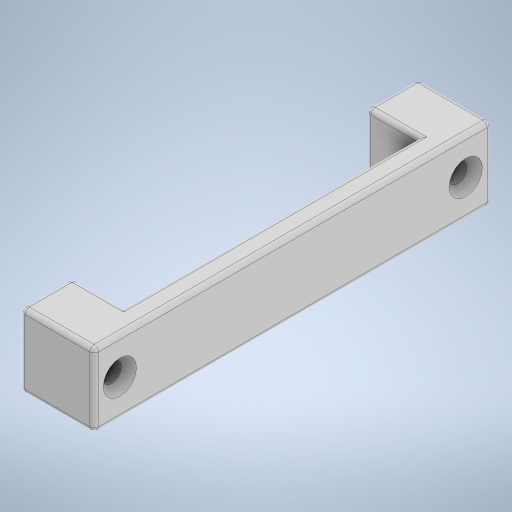
# Autodesk Inventor part: PMSretainer
Saved by Autodesk Inventor 2024 (Build 280153000, 153)
## iProperties
Created: 2023-11-03
Part Number: PMSretainer
Material: Generic
Document SubType Name: Modeling
Designer: njspada
Density: 1 g/cm^3
Appearance: Default
Author: njspada
Autodesk Inventor part; units mm, degrees
ref_plane "YZ Plane" through (0, 0, 0) normal (1, 0, 0) x (0, 1, 0)
ref_plane "XZ Plane" through (0, 0, 0) normal (0, 1, 0) x (-1, 0, 0)
ref_plane "XY Plane" through (0, 0, 0) normal (0, 0, 1) x (1, 0, 0)
sketch "Sketch1" plane through (0, 0, 0) normal (0, 1, 0) x (-1, 0, 0)
  line L0 (0, 0) -> (3.81, 0)
  line L1 (3.81, 0) -> (3.81, -50.8)
  line L2 (3.81, -50.8) -> (0, -50.8)
  line L3 (0, -50.8) -> (0, 0)
  line L4 (0, 0) -> (12.7, 0)
  line L5 (12.7, 0) -> (12.7, 8.89)
  line L6 (12.7, 8.89) -> (0, 8.89)
  line L7 (0, 8.89) -> (0, 0)
  line L8 (0, -50.8) -> (12.7, -50.8)
  line L9 (12.7, -50.8) -> (12.7, -59.69)
  line L10 (12.7, -59.69) -> (0, -59.69)
  line L11 (0, -59.69) -> (0, -50.8)
  dimension "d0" = 3.81
  dimension "d1" = 50.8
  dimension "d2" = 12.7
  dimension "d3" = 8.89
  dimension "d4" = 12.7
  dimension "d5" = 8.89
  constraints: 24 end point, 6 parallel, 3 horizontal, 3 perpendicular
  measures "d0" distance of L1.end L2.end
  measures "d1" distance of L0.end L1.end
  measures "d2" distance of L6.end L5.end
  measures "d3" distance of L5.end L4.end
  measures "d4" distance of L9.end L10.end
  measures "d5" distance of L8.end L9.end
extrude "Extrusion1" add sketch "Sketch1" along normal blind 12.7
sketch "Sketch2" plane through (0, 0, 8.89) normal (1, 0, 0) x (0, 0, -1)
  line L0 (0, 12.7) -> (68.58, 12.7) construction
  line L1 (8.89, 0) -> (0, 0) construction
  line L2 (0, 0) -> (0, 12.7) construction
  line L3 (0, 12.7) -> (8.89, 12.7) construction
  line L4 (8.89, 12.7) -> (8.89, 0) construction
  line L5 (34.29, 12.7) -> (34.29, 0) construction
  line L6 (59.69, 0) -> (8.89, 0) construction
  point P0 (4.445, 6.35)
  point P1 (64.135, 6.35)
  constraints: 10 end point, 2 midpoint, 2 parallel, 1 horizontal, 1 perpendicular, 1 symmetric about line
hole "Hole1" at (0, 6.35, 4.445) at (0, 6.35, -55.245) direction (-1, 0, 0) diameter 3.2766 end through all countersink diameter 5.715 countersink angle 82 clearance for "Flat Head Machine Screw (82)" size "#4" standard "Ansi Unified Screw Threads"
fillet "Fillet1" radius 0.762 24 edges at (-6.35, 12.7, 8.89) (-6.35, 0, 8.89) (0, 6.35, 8.89) (0, 12.7, -25.4) (0, 0, -25.4) (0, 6.35, -59.69) (-8.255, 12.7, 0) (-3.81, 12.7, -25.4) (-8.255, 12.7, -50.8) (-12.7, 12.7, 4.445) (-12.7, 6.35, 8.89) (-6.35, 12.7, -59.69) (-6.35, 0, -59.69) (-8.255, 0, -50.8) (-8.255, 0, 0) (-3.81, 0, -25.4) (-12.7, 6.35, -50.8) (-12.7, 6.35, -59.69) (-12.7, 6.35, -53.6067) (-12.7, 12.7, -55.245) (-12.7, 0, -55.245) (-12.7, 0, 4.445) (-12.7, 6.35, 0) (-12.7, 6.35, 6.0833)
body "Solid1"
